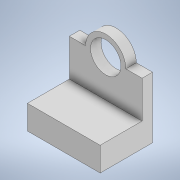
# Autodesk Inventor part: exercise2
Saved by Autodesk Inventor 2020 (Build 240168000, 168)
## iProperties
Created: 2021-11-12
Part Number: exercise2
Material: Generic
Document SubType Name: Modeling
Designer: rwte
Density: 1 g/cm^3
Appearance: Default
Author: rwte
Autodesk Inventor part; units mm, degrees
ref_plane "YZ Plane" through (0, 0, 0) normal (1, 0, 0) x (0, 1, 0)
ref_plane "XZ Plane" through (0, 0, 0) normal (0, 1, 0) x (-1, 0, 0)
ref_plane "XY Plane" through (0, 0, 0) normal (0, 0, 1) x (1, 0, 0)
sketch "Sketch1" plane through (0, 0, 0) normal (0, 0, 1) x (1, 0, 0)
  line L0 (-6.9396, 11.6683) -> (6.9396, 11.6683)
  line L1 (6.9396, 11.6683) -> (6.9396, 0)
  line L2 (6.9396, 0) -> (-6.9396, 0)
  line L3 (-6.9396, 0) -> (-6.9396, 11.6683)
  circle A0 centre (0, 11.6683) radius 3.8335
  circle A1 centre (0, 11.6683) radius 2.9035
  point P0 (0, 0)
  point P1 (0, 0)
  point P2 (3.8335, 11.6683)
  point P3 (-3.8335, 11.6683)
  constraints: 8 end point, 2 centre point, 2 coincident, 2 midpoint, 2 parallel, 1 horizontal, 1 perpendicular
extrude "Extrusion1" add sketch "Sketch1" along normal blind 2 contours A1 L0 A0 | L0 A0 A1 | L0 L1 L2 L3 A0
sketch "Sketch2" plane through (0, 0, 0) normal (0, 0, 1) x (1, 0, 0)
  line L0 (-6.9396, 11.6683) -> (-6.9396, 0) projected
  line L1 (-6.9396, 0) -> (6.9396, 0)
  line L2 (6.9396, 0) -> (6.9396, 4.5855)
  line L3 (6.9396, 4.5855) -> (-6.9396, 4.5855)
  line L4 (-6.9396, 4.5855) -> (-6.9396, 0)
  line L5 (6.9396, 0) -> (6.9396, 11.6683) projected
  point P0 (0, 0)
  constraints: 8 end point, 2 parallel, 1 horizontal, 1 perpendicular, 1 point on line
extrude "Extrusion2" add sketch "Sketch2" along normal blind 10
body "Solid1"
